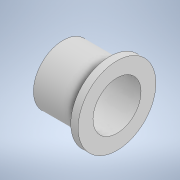
# Autodesk Inventor part: pipeForFrontPipeDrain
Saved by Autodesk Inventor 2021.1 (Build 251245010, 245A)
## iProperties
Created: 2020-10-20
Part Number: pipeForFrontPipeDrain
Material: Generic
Document SubType Name: Modeling
Designer: robst
Density: 1 g/cm^3
Appearance: Default
Author: robst
Autodesk Inventor part; units mm, degrees
ref_plane "YZ Plane" through (0, 0, 0) normal (1, 0, 0) x (0, 1, 0)
ref_plane "XZ Plane" through (0, 0, 0) normal (0, 1, 0) x (-1, 0, 0)
ref_plane "XY Plane" through (0, 0, 0) normal (0, 0, 1) x (1, 0, 0)
sketch "Sketch2" plane through (0, 0, 0) normal (0, 0, 1) x (1, 0, 0)
  line L0 (0, 0) -> (0, 15.875)
  line L1 (0, 15.875) -> (-2.9977, 15.875)
  line L2 (-2.9977, 15.875) -> (-2.9977, 12.0714)
  line L3 (-2.9977, 12.0714) -> (-22.0477, 12.0714)
  line L4 (-22.0477, 12.0714) -> (-22.0477, 9.815)
  line L5 (-22.0477, 9.815) -> (0, 9.815)
  line L6 (-26.4573, 0) -> (4.4095, 0) projected
  dimension "d0" = 15.875
  dimension "d1" = 9.815
  dimension "d2" = 2.9977
  dimension "d3" = 19.05
  constraints: 12 end point, 5 perpendicular, 1 point on line, 1 vertical
  measures "d0" distance from line of L0.start L1
  measures "d1" distance from line of L5 L0.start
  measures "d2" distance between parallel lines of L0 L2
  measures "d3" distance from line of L3.end L2
revolve "Revolution1" add sketch "Sketch2" angle 360 about axis through (-10, 0, 0) along (1, 0, 0)
equation "\"d0\" = outsideRadius"
equation "\"d3\" = houseWallThickness"
equation "\"outsideDiameter\" = 31.75"
equation "\"pipeDiameter\" = 26.67"
equation "\"outsideRadius\" = 0.5 * outsideDiameter"
equation "\"pipeRadius\" = 0.5 * pipeDiameter"
equation "\"wallThickness\" = 3.175"
equation "\"houseWallThickness\" = 19.05"
body "Solid1"
